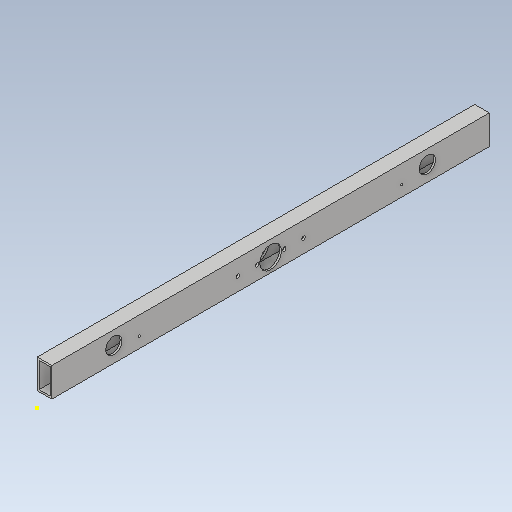
# Autodesk Inventor part: 2x1 20in Alluminum with Cal Drop.ver1-1111-2019
Saved by Autodesk Inventor 2020 (Build 240168000, 168)
## iProperties
Created: 2019-10-10
Part Number: 2x1 20in Alluminum with Cal Drop.ver1-1111-2019
Material: Generic
Document SubType Name: Modeling
Designer: JMHal
Density: 1 g/cm^3
Appearance: Default
Author: JMHal
Autodesk Inventor part; units mm, degrees
ref_plane "YZ Plane" through (0, 0, 0) normal (1, 0, 0) x (0, 1, 0)
ref_plane "XZ Plane" through (0, 0, 0) normal (0, 1, 0) x (-1, 0, 0)
sketch "Sketch1" plane through (0, 0, 0) normal (0, 1, 0) x (-1, 0, 0)
  point P0 (0, 0)
sketch "Sketch2" plane through (0, 0, 0) normal (0, 1, 0) x (-1, 0, 0)
  line L0 (0, 0) -> (25.4, 0)
  line L1 (25.4, 0) -> (25.4, -812.8)
  line L2 (25.4, -812.8) -> (0, -812.8)
  line L3 (0, -812.8) -> (0, 0)
  dimension "d0" = 812.8
  dimension "d1" = 25.4
  constraints: 8 end point, 2 parallel, 1 horizontal, 1 perpendicular
  measures "d0" distance of L0.end L1.end
  measures "d1" distance of L1.end L2.end
extrude "Extrusion1" add sketch "Sketch2" along normal blind 50.8
sketch "Sketch3" plane through (0, 0, 0) normal (1, 0, 0) x (0, 0, -1)
  circle A0 centre (133.35, 26.9875) radius 14.2875
  line L0 (0, 0) -> (0, 50.8) projected
  line L1 (0, 50.8) -> (812.8, 50.8) projected
  circle A1 centre (679.45, 26.9875) radius 14.2875
  line L2 (812.8, 0) -> (812.8, 50.8) projected
  line L3 (812.8, 0) -> (0, 0) projected
  circle A2 centre (406.4, 23.8125) radius 19.05
  point P0 (406.4, 50.8)
  point P1 (406.4, 0)
  point P2 (406.4, 0)
  dimension "d4" = 28.575
  dimension "d5" = 133.35
  dimension "d6" = 23.8125
  dimension "d7" = 28.575
  dimension "d8" = 133.35
  dimension "d9" = 26.9875
  dimension "d10" = 38.1
  dimension "d11" = 26.9875
  constraints: 3 centre point, 3 midpoint, 3 vertical alignment
  measures "d4" diameter of A0
  measures "d5" distance from line of A0.centre L0
  measures "d6" distance from line of A0.centre L1
  measures "d7" diameter of A1
  measures "d8" distance from line of L2 A1.centre
  measures "d9" distance from line of A1.centre L3
  measures "d10" diameter of A2
  measures "d11" distance from line of A2.centre L1
extrude "Extrusion2" cut sketch "Sketch3" against normal through all contours A0 | A1 | A2
sketch "Sketch4" plane through (-25.4, 0, 0) normal (0, 0, 1) x (1, 0, 0)
  line L0 (0, 50.8) -> (25.4, 50.8) projected
  line L1 (25.4, 0) -> (25.4, 50.8) projected
  line L2 (25.4, 0) -> (0, 0) projected
  line L3 (0, 0) -> (0, 50.8) projected
  line L4 (22.225, 47.625) -> (3.175, 47.625)
  line L5 (3.175, 47.625) -> (3.175, 3.175)
  line L6 (3.175, 3.175) -> (22.225, 3.175)
  line L7 (22.225, 3.175) -> (22.225, 47.625)
  dimension "d15" = 3.175
  constraints: 8 end point, 3 other
  measures "d15" distance between parallel lines of L0 L4
extrude "Extrusion3" cut sketch "Sketch4" against normal up to surface (812.8 mm away) contours L7 L6 L5 L4
sketch "Sketch5" plane through (0, 0, 0) normal (1, 0, 0) x (0, 0, -1)
  circle A0 centre (679.45, 26.9875) radius 14.2875 projected
  circle A1 centre (133.35, 26.9875) radius 14.2875 projected
  circle A2 centre (406.4, 23.8125) radius 19.05 projected
  line L0 (812.8, 0) -> (0, 0) projected
  line L1 (812.8, 0) -> (812.8, 50.8) projected
  line L2 (0, 50.8) -> (812.8, 50.8) projected
  line L3 (0, 0) -> (0, 50.8) projected
  line L4 (0, 50.8) -> (25.4, 50.8)
  line L5 (25.4, 50.8) -> (25.4, 0)
  line L6 (25.4, 0) -> (0, 0)
  line L7 (0, 0) -> (0, 50.8)
  line L8 (812.8, 0) -> (812.8, 50.8) projected
  line L9 (812.8, 0) -> (0, 0) projected
  line L10 (812.8, 50.8) -> (787.4, 50.8)
  line L11 (787.4, 50.8) -> (787.4, 0)
  line L12 (787.4, 0) -> (812.8, 0)
  line L13 (812.8, 0) -> (812.8, 50.8)
  dimension "d18" = 25.4
  dimension "d19" = 25.4
  dimension "d59" = 28.575
  constraints: 16 end point, 4 parallel, 2 horizontal, 2 perpendicular, 2 point on line
  measures "d18" distance between parallel lines of L3 L5
  measures "d19" distance between parallel lines of L1 L11
  measures "d59" diameter of A0
extrude "Extrusion4" cut sketch "Sketch5" against normal blind 25.4 contours L0 L11 L2 L1 | L0 L3 L2 L5
sketch "Sketch8" plane through (0, 0, -25.4) normal (1, 0, 0) x (0, 0, -1)
  point P0 (-25.4, 0)
sketch "Sketch9" plane through (0, 0, -25.4) normal (1, 0, 0) x (0, 0, -1)
  circle A0 centre (404.8252, 23.8125) radius 3.175
  circle A1 centre (381, 23.8125) radius 19.05 projected
  line L0 (0, 50.8) -> (762, 50.8) projected
  circle A2 centre (357.1748, 23.8125) radius 3.175
  circle A3 centre (438.1754, 23.8125) radius 3.175
  circle A4 centre (323.8246, 23.8125) radius 3.175
  point P0 (-25.4, 0)
  point P1 (257.298, 23.8125)
  dimension "d61" = 6.35
  dimension "d62" = 23.8252
  dimension "d64" = 6.35
  dimension "d65" = 23.8252
  dimension "d67" = 6.35
  dimension "d69" = 6.35
  dimension "d71" = 57.1754
  dimension "d72" = 57.1754
  constraints: 4 centre point, 4 horizontal alignment
  measures "d61" diameter of A0
  measures "d62" distance of A0.centre A1.centre
  measures "d64" diameter of A2
  measures "d65" distance of A1.centre A2.centre
  measures "d67" diameter of A3
  measures "d69" diameter of A4
  measures "d71" distance of A1.centre A4.centre
  measures "d72" distance of A3.centre A1.centre
extrude "Extrusion6" cut sketch "Sketch9" against normal blind 25.4 contours A0 | A2 | A3 | A4
sketch "Sketch11" plane through (-25.4, 0, -787.4) normal (-1, 0, 0) x (0, 0, 1)
  circle A0 centre (438.1754, 23.8125) radius 4.7625
  circle A1 centre (381, 23.8125) radius 19.05 projected
  line L0 (0, 50.8) -> (762, 50.8) projected
  circle A2 centre (323.8246, 23.8125) radius 4.7625
  point P0 (787.4, 0)
  dimension "d85" = 9.525
  dimension "d86" = 57.1754
  dimension "d88" = 9.525
  dimension "d90" = 57.1754
  constraints: 2 centre point, 2 horizontal alignment
  measures "d85" diameter of A0
  measures "d86" distance of A0.centre A1.centre
  measures "d88" diameter of A2
  measures "d90" distance of A1.centre A2.centre
extrude "Extrusion8" cut sketch "Sketch11" against normal blind 12.7 contours A0 | A2
sketch "Sketch12" plane through (-25.4, 0, -787.4) normal (-1, 0, 0) x (0, 0, 1)
  circle A0 centre (609.6, 19.05) radius 4.7625
  line L0 (762, 0) -> (0, 0) projected
  circle A1 centre (381, 23.8125) radius 19.05 projected
  circle A2 centre (654.05, 26.9875) radius 14.2875 projected
  point P0 (787.4, 0)
  dimension "d93" = 9.525
  dimension "d94" = 19.05
  dimension "d103" = 44.45
  constraints: 1 centre point
  measures "d93" diameter of A0
  measures "d94" distance from line of A0.centre L0
  measures "d103" horizontal distance of A2.centre A0.centre
extrude "Extrusion9" cut sketch "Sketch12" against normal blind 12.7 contours A0
sketch "Sketch13" plane through (0, 0, -25.4) normal (1, 0, 0) x (0, 0, -1)
  circle A0 centre (152.4, 19.05) radius 1.905
  circle A1 centre (381, 23.8125) radius 19.05 projected
  line L0 (762, 0) -> (0, 0) projected
  circle A2 centre (107.95, 26.9875) radius 14.2875 projected
  point P0 (-25.4, 0)
  dimension "d98" = 3.81
  dimension "d100" = 19.05
  dimension "d104" = 44.45
  constraints: 1 centre point
  measures "d98" diameter of A0
  measures "d100" distance from line of L0 A0.centre
  measures "d104" horizontal distance of A2.centre A0.centre
extrude "Extrusion10" cut sketch "Sketch13" against normal blind 12.7 contours A0
ref_plane "Work Plane1" through (0, 0, -406.4) normal (0, 0, 1) x (1, 0, 0)
mirror "Mirror1" about plane through (0, 0, -406.4) normal (0, 0, 1) of "Extrusion10", "Extrusion9"
equation "\"d9\" = d11"
body "Solid1"
